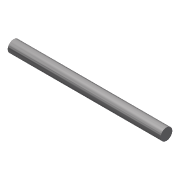
# Autodesk Inventor part: Top_Arm_Rod
Saved by Autodesk Inventor 2016 (Build 200138000, 138)
## iProperties
Created: 2015-05-19
Part Number: Top_Arm_Rod
Material: Stainless Steel
Document SubType Name: Modeling
Designer: CHUNGBK
Density: 8 g/cm^3
Appearance: Semi-Polished
Mass: 125.486 g
Surface Area: 51.9375 cm^2
Volume: 15.6858 cm^3
Author: CHUNGBK
Autodesk Inventor part; units mm, degrees
ref_plane "YZ Plane" through (0, 0, 0) normal (1, 0, 0) x (0, 1, 0)
ref_plane "XZ Plane" through (0, 0, 0) normal (0, 1, 0) x (-1, 0, 0)
ref_plane "XY Plane" through (0, 0, 0) normal (0, 0, 1) x (1, 0, 0)
sketch "Sketch1" plane through (0, 0, 0) normal (1, 0, 0) x (0, 1, 0)
  circle A0 centre (0, 0) radius 4.7625
  dimension "d0" = 9.525
  constraints: 1 centre point, 1 coincident
  measures "d0" diameter of A0
extrude "Extrusion1" add sketch "Sketch1" along normal blind 123.825
body "Solid1"
